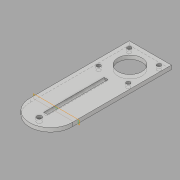
# Autodesk Inventor part: DispenserBrace
Saved by Autodesk Inventor 2017 (Build 210142000, 142)
## iProperties
Created: 2017-05-24
Part Number: DispenserBrace
Material: Generic
Document SubType Name: Modeling
Designer: gmarsh
Density: 1 g/cm^3
Appearance: Default
Author: gmarsh
Autodesk Inventor part; units mm, degrees
ref_plane "YZ Plane" through (0, 0, 0) normal (1, 0, 0) x (0, 1, 0)
ref_plane "XY Plane" through (0, 0, 0) normal (0, 0, 1) x (1, 0, 0)
sketch "Sketch1" plane through (0, 0, 0) normal (0, 0, 1) x (1, 0, 0)
  line L0 (-22, 38.0007) -> (21.9822, 38.0007)
  line L1 (21.9822, 38.0007) -> (21.9822, -66)
  line L2 (-22, -66) -> (-22, 38.0007)
  arc A0 (-22, -65.3741) -> (21.9822, -65.3741) centre (-0.0089, -66) ccw
  point P0 (0, 0)
  dimension "d22" = 44
  constraints: 6 end point, 2 point on circle, 2 point on line, 2 vertical, 1 centre point
  measures "d22" diameter of A0
extrude "Extrusion1" add sketch "Sketch1" along normal blind 4
sketch "Sketch2" plane through (0, 0, 0) normal (0, 0, 1) x (1, 0, 0)
  circle A0 centre (-15.5, 31.5) radius 2
  circle A1 centre (15.5, 31.5) radius 2
  circle A2 centre (-15.5, -0.5) radius 2
  circle A3 centre (15.5, -0.5) radius 2
  point P0 (0, 0)
  constraints: 4 centre point
extrude "Extrusion2" cut sketch "Sketch2" along normal blind 4
sketch "Sketch3" plane through (0, 0, 0) normal (0, 0, 1) x (1, 0, 0)
  circle A0 centre (0, -78) radius 2.5
  point P0 (0, 0)
  dimension "d24" = 5
  constraints: 1 centre point
  measures "d24" diameter of A0
extrude "Extrusion3" cut sketch "Sketch3" along normal blind 4
ref_plane "Work Plane1" through (0, -60, 0) normal (0, 1, 0) x (-1, 0, 0)
sketch "Sketch4" plane through (0, -60, 0) normal (0, 1, 0) x (-1, 0, 0)
  circle A0 centre (0, 4) radius 2
  point P0 (0, 0)
  dimension "d14" = 4
  constraints: 1 centre point
  measures "d14" diameter of A0
extrude "Extrusion4" cut sketch "Sketch4" along normal blind 51.75 and the other way blind 11.25
sketch "Sketch5" plane through (0, 0, 4) normal (0, 0, 1) x (1, 0, 0)
  circle A0 centre (0, 16.6667) radius 12.5
  point P0 (0, 0)
  dimension "d19" = 25
  constraints: 1 centre point
  measures "d19" diameter of A0
extrude "Extrusion5" cut sketch "Sketch5" against normal blind 4
body "Solid1"
